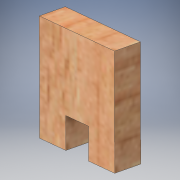
# Autodesk Inventor part: Tope para Motor Prototipo Inicial
Saved by Autodesk Inventor 2016 SP2 (Build 200236200, 236)
## iProperties
Created: 2017-06-26
Part Number: Tope para Motor Prototipo Inicial
Material: Abedul
Document SubType Name: Modeling
Designer: ssant
Density: 0.512 g/cm^3
Appearance: Abedul - Natural brillo medio
Author: ssant
Autodesk Inventor part; units mm, degrees
ref_plane "YZ Plane" through (0, 0, 0) normal (1, 0, 0) x (0, 1, 0)
ref_plane "XZ Plane" through (0, 0, 0) normal (0, 1, 0) x (-1, 0, 0)
ref_plane "XY Plane" through (0, 0, 0) normal (0, 0, 1) x (1, 0, 0)
sketch "Boceto1" plane through (0, 0, 0) normal (0, 0, 1) x (1, 0, 0)
  line L0 (15, -17.5) -> (15, 17.5)
  line L1 (15, 17.5) -> (-15, 17.5)
  line L2 (-15, 17.5) -> (-15, -17.5)
  line L3 (-15, -17.5) -> (-5, -17.5)
  line L4 (5, -17.5) -> (15, -17.5)
  line L5 (-4.5, -17.5) -> (-4.5, -7.5)
  line L6 (-4.5, -7.5) -> (4.5, -7.5)
  line L7 (4.5, -7.5) -> (4.5, -17.5)
  line L8 (-4.5, -17.5) -> (-5, -17.5)
  line L9 (4.5, -17.5) -> (5, -17.5)
  point P0 (0, 0)
  point P1 (15, 0)
  point P2 (0, -7.5)
  point P3 (0, -17.5)
  dimension "d0" = 30
  dimension "d1" = 35
  dimension "d7" = 10
  dimension "d8" = 9
  dimension "d9" = 15
  constraints: 20 end point, 4 perpendicular, 3 horizontal, 3 parallel, 2 midpoint, 1 collinear, 1 horizontal alignment, 1 point on line, 1 vertical, 1 vertical alignment
  measures "d0" distance of L1.end L0.end
  measures "d1" distance of L0.end L0.start
  measures "d7" distance of L5.start L5.end
  measures "d8" distance of L5.end L6.end
  measures "d9" distance from line of L0 point (0, -7.5)
extrude "Extrusión2" add sketch "Boceto1" along normal blind 9
